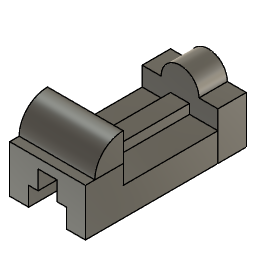
Robocon Task 1-2 (Autodesk Fusion 360 design; units mm, degrees)
Autodesk Fusion 360 part; units mm, degrees
sketch "Sketch1" plane through (0, 0, 0) normal (1, 0, 0) x (0, 1, 0)
  line L0 (0, 0, 0) -> (0, 0, 10)
  line L1 (0, 0) -> (0, 25)
  line L2 (0, 25, 0) -> (0, 25, 40)
  line L3 (0, 25, 40) -> (0, 0, 40)
  line L4 (0, 0, 40) -> (0, 0, 30)
  line L5 (0, 0, 30) -> (0, 10, 30)
  line L6 (0, 10, 30) -> (0, 10, 25)
  line L7 (0, 10, 25) -> (0, 20, 25)
  line L8 (0, 20, 25) -> (0, 20, 15)
  line L9 (0, 20, 15) -> (0, 10, 15)
  line L10 (0, 10, 15) -> (0, 10, 10)
  line L11 (0, 10, 10) -> (0, 0, 10)
  dimension "d8" = 10
  dimension "d9" = 25
  dimension "d10" = 40
  dimension "d11" = 25
  dimension "d12" = 10
  dimension "d13" = 10
  dimension "d14" = 5
  dimension "d15" = 10
  dimension "d16" = 10
  dimension "d17" = 10
  dimension "d18" = 5
  constraint coincident L1.start origin
  constraint vertical L1
  measures "d8" distance of L1.start origin
  measures "d9" distance of L1.start L1.end
  measures "d11" distance of L1.end L1.start
  measures "d12" distance of L1.start origin
extrude "Extrude1" add sketch "Sketch1" along normal blind 20 contours L0 L1 L2 L3 L4 L5 L6 L7 L8 L9 L10 L11 in plane through (0, 0, 0) normal (0, 1, 0) makes body 1
sketch "Sketch2" plane through (40, 0, 0) normal (1, 0, 0) x (0, 1, 0)
  line L0 (0, 25) -> (0, 0)
  line L1 (0, 0) -> (20, 0)
  line L2 (20, 0) -> (20, 25)
  line L3 (20, 25) -> (0, 25)
  line L4 (20, 0) -> (20, 15)
  line L5 (20, 0, -40) -> (20, 0, -30)
  line L6 (20, 0, 0) -> (20, 0, -10)
  line L7 (20, 0, -10) -> (20, 10, -10)
  line L8 (20, 10, -10) -> (20, 10, -15)
  line L9 (20, 10, -30) -> (20, 0, -30)
  line L10 (20, 0) -> (20, 15)
  line L11 (20, 15, 0) -> (20, 15, -10)
  line L12 (20, 10, -15) -> (20, 20, -15)
  line L13 (20, 15, -10) -> (20, 15, -15)
  line L14 (20, 15, -15) -> (20, 20, -15)
  line L15 (20, 0, -40) -> (20, 15, -40)
  line L16 (20, 20, -25) -> (20, 10, -25)
  line L17 (20, 15, -40) -> (20, 15, -25)
  line L18 (20, 15, -25) -> (20, 10, -25)
  line L19 (20, 10, -25) -> (20, 10, -30)
  point P0 (20, 0)
  point P1 (20, 0)
  point P2 (20, 0)
  point P3 (20, 10)
  point P4 (20, 10)
  point P5 (20, 10)
  point P6 (20, 10)
  dimension "d21" = 15
  dimension "d30" = 5
  dimension "d31" = 15
  dimension "d32" = 15
  constraint coincident P2 P1
  constraint perpendicular L1 L4
  constraint coincident P6 P5
  constraint perpendicular L1 L10
  measures "d21" distance of P2 L4.end
  measures "d30" distance of P6 L4.end
  measures "d31" distance of P2 L4.end
  measures "d32" distance of P2 L4.end
sketch "Sketch3" plane through (0, 20, 0) normal (0, 1, 0) x (-1, 0, 0)
  line L0 (0, 0) -> (0, 25)
  line L1 (0, 25) -> (-40, 25)
  line L2 (-40, 25) -> (-40, 0)
  line L3 (-40, 0) -> (-30, 0)
  line L4 (-30, 0) -> (-30, 10)
  line L5 (-30, 10) -> (-25, 10)
  line L6 (-25, 10) -> (-25, 20)
  line L7 (-25, 20) -> (-15, 20)
  line L8 (-15, 20) -> (-15, 10)
  line L9 (-15, 10) -> (-10, 10)
  line L10 (-10, 10) -> (-10, 0)
  line L11 (-10, 0) -> (0, 0)
  line L12 (-25, 10) -> (-25, 15)
  line L13 (-15, 10) -> (-15, 15)
  line L14 (-25, 10) -> (-25.0023, 14.7352)
  point P0 (-25.0023, 14.7352)
  point P1 (-15.0023, 14.7352)
  dimension "d27" = 5
  dimension "d29" = 5
  constraint coincident L5.end L6.start
  constraint perpendicular L5 L12
  constraint coincident L8.end L9.start
  constraint perpendicular L9 L13
  constraint coincident P0 L14.end
  measures "d27" distance of L5.end L12.end
  measures "d29" distance of L8.end L13.end
extrude "Extrude2" add sketch "Sketch2" along normal blind 50 contours L5 L9 L15 L16 L17 L18 L19 in plane through (40, 20, 0) normal (0, 1, 0) bodies 1
sketch "Sketch4" plane through (40, 0, 0) normal (1, 0, 0) x (0, 1, 0)
  line L0 (0, 25) -> (0, 0)
  line L1 (0, 0) -> (20, 0)
  line L2 (20, 0) -> (20, 25)
  line L3 (20, 25) -> (0, 25)
  line L4 (20, 10, -15) -> (20, 15, -15)
  line L5 (20, 15, -15) -> (20, 15.001, 0)
  line L6 (20, 10, -15) -> (20, 10, -10)
  line L7 (20, 10, -10) -> (20, 0, -10)
  line L8 (20, 0, -10) -> (20, 0, 0)
  point P0 (20, 14.7352)
  point P1 (20, 10)
  point P2 (20, 15)
  dimension "d37" = 15
  dimension "d38" = 5
  dimension "d39" = 10
  dimension "d40" = 10
  measures "d39" distance of P1 L1.end
  measures "d40" distance of L1.end L2.start
extrude "Extrude3" add sketch "Sketch4" along normal blind 50 contours L2 L4 L5 L6 L7 L8 in plane through (40, 20, 0) normal (0, 1, 0) bodies 1
sketch "Sketch5" plane through (0, 20, 0) normal (0, 1, 0) x (-1, 0, 0)
  line L0 (-40, 15.001) -> (-25, 15)
  line L1 (-25, 15) -> (-25, 20)
  line L2 (-25, 20) -> (-15, 20)
  line L3 (-15, 20) -> (-15, 15)
  line L4 (-15, 15) -> (0, 15)
  line L5 (0, 15) -> (0, 25)
  line L6 (0, 25) -> (-40, 25)
  line L7 (-40, 25) -> (-40, 15.001)
  line L8 (-25, 15) -> (-25, 20)
  line L9 (-25, 20) -> (-15, 20)
  line L10 (-15, 20) -> (-15, 15)
  constraint coincident L0.end L1.start
  constraint perpendicular L2 L8
  constraint coincident L2.end L3.start
  constraint coincident L3.end L4.start
sketch "Sketch6" plane through (0, 0, 15) normal (0, 0, 1) x (-1, 0, 0)
  line L0 (0, -20) -> (-15, -20)
  line L1 (-15, -20) -> (-15, -70)
  line L2 (-15, -70) -> (0, -70)
  line L3 (0, -70) -> (0, -20)
  line L4 (-25, -20) -> (-15, -20)
  line L5 (-15, -20, 0) -> (-15, -20, 5)
  line L6 (-15, -20, 5) -> (-25, -20, 5)
  line L7 (-25, -20, 5) -> (-25, -20, 0)
  point P0 (-25, -20)
  point P1 (-15, -20)
  point P2 (-25, -20)
  constraint coincident P2 P0
  constraint coincident P1 L0.end
extrude "Extrude4" add sketch "Sketch6" against normal blind 50 contours L4 L5 L6 L7 in plane through (0, 20, 15) normal (0, -1, 0) bodies 1
sketch "Sketch7" plane through (0, 70, 0) normal (0, 1, 0) x (-1, 0, 0)
  line L0 (-30, 10) -> (-25, 10)
  line L1 (-25, 10) -> (-25, 15)
  line L2 (-40, 15.001) -> (-40, 0)
  line L3 (-40, 0) -> (-30, 0)
  line L4 (-30, 0) -> (-30, 10)
  line L5 (-40, 0) -> (-40, 25)
  line L6 (-40, 25) -> (-30, 25)
  arc A0 (-10, 25) -> (-30, 25) centre (-20, 25) ccw
  line L7 (-10, 25) -> (0, 25)
  line L8 (0, 25) -> (0, 15)
  line L9 (0, 15) -> (0, 0)
  line L10 (0, 0) -> (-10, 0)
  line L11 (-10, 0) -> (-10, 10)
  line L12 (-10, 10) -> (-15, 10)
  line L13 (-15, 10) -> (-15, 15)
  line L14 (-15, 15) -> (-25, 15)
  line L15 (-25, 10) -> (-30, 10)
  line L16 (-25, 15) -> (-25, 10)
  line L17 (-30, 10) -> (-30, 0)
  line L18 (-30, 0) -> (-40, 0)
  point P0 (0, 15)
  point P1 (-10, 0)
  point P2 (-10, 10)
  point P3 (-15, 10)
  point P4 (-15, 15)
  dimension "d46" = 25
  dimension "d48" = 10
  dimension "d49" = 10
  dimension "d50" = 10
  constraint coincident L2.end L3.start
  constraint perpendicular L3 L5
  constraint perpendicular L5 L6
  constraint horizontal L7
  constraint coincident P0 L8.end
  constraint perpendicular L7 L8
  constraint coincident L9.end L10.start
  constraint coincident P1 L10.end
  constraint coincident P2 L11.end
  constraint coincident P3 L12.end
  constraint coincident P4 L13.end
  constraint coincident L1.end L14.end
  constraint coincident L0.end L1.start
  constraint coincident L0.start L4.end
  constraint coincident L3.end L4.start
  measures "d46" distance of L2.end L5.end
  measures "d48" distance of L6.end A0.centre
  measures "d49" radius of A0
  measures "d50" distance of A0.start L7.end
extrude "Extrude5" add sketch "Sketch7" along normal blind 15 separate body makes body 2
sketch "Sketch8" plane through (40, 0, 0) normal (1, 0, 0) x (0, 1, 0)
  line L0 (0, 25) -> (0, 0)
  line L1 (0, 0) -> (70, 0)
  line L2 (70, 0) -> (70, 15.001)
  line L3 (70, 15.001) -> (20, 15.001)
  line L4 (20, 15.001) -> (20, 25)
  line L5 (20, 25) -> (0, 25)
  arc A0 (20, 40) -> (5, 25) centre (20, 25) ccw
  line L6 (20, 25) -> (20, 40) construction
  line L7 (20, 25) -> (5, 25) construction
  line L8 (5, 25) -> (20, 25)
  line L9 (20, 40) -> (20, 25)
  constraint coincident L4.end L5.start
  constraint perpendicular L6 L8
extrude "Extrude6" add sketch "Sketch8" against normal blind 40 separate body contours L5 A0 L8 L9 makes body 3
